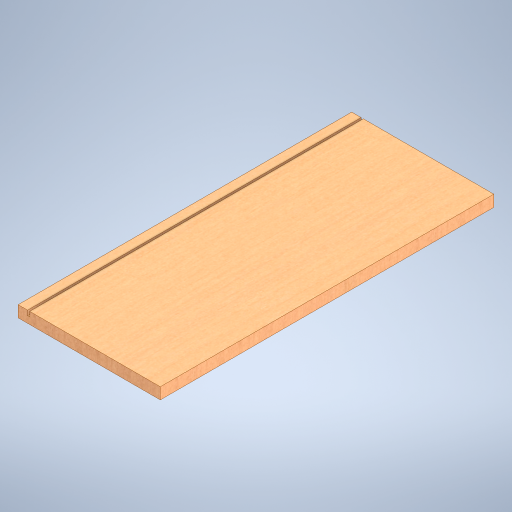
# Autodesk Inventor part: Querseite_Shotclock
Saved by Autodesk Inventor 2024 (Build 280153000, 153)
## iProperties
Created: 2024-03-12
Part Number: Querseite_Shotclock
Material: Holz (Kirsche)
Document SubType Name: Modeling
Designer: haniv
Density: 0.63 g/cm^3
Appearance: Kirsche - natur - schwacher Glanz
Author: haniv
Autodesk Inventor part; units mm, degrees
ref_plane "YZ Plane" through (0, 0, 0) normal (1, 0, 0) x (0, 1, 0)
ref_plane "XZ Plane" through (0, 0, 0) normal (0, 1, 0) x (-1, 0, 0)
ref_plane "XY Plane" through (0, 0, 0) normal (0, 0, 1) x (1, 0, 0)
sketch "Skizze1" plane through (0, 0, 0) normal (0, 0, 1) x (1, 0, 0)
  line L0 (-75, 176) -> (75, 176)
  line L1 (75, 176) -> (75, -176)
  line L2 (75, -176) -> (-75, -176)
  line L3 (-75, -176) -> (-75, 176)
  point P0 (0, 0)
  point P1 (0, 176)
  point P2 (-75, 0)
  dimension "d0" = 150
  dimension "d1" = 352
  constraints: 8 end point, 2 midpoint, 2 parallel, 1 horizontal, 1 horizontal alignment, 1 perpendicular, 1 vertical alignment
  measures "d0" distance of L1.end L2.end
  measures "d1" distance of L0.end L1.end
extrude "Extrusion1" add sketch "Skizze1" along normal blind 12
sketch "Skizze2" plane through (0, 0, 12) normal (0, 0, 1) x (1, 0, 0)
  line L0 (-75, -176) -> (75, -176) projected
  line L1 (75, -176) -> (75, 176) projected
  line L2 (75, 176) -> (-75, 176) projected
  line L3 (-75, 176) -> (-75, -176) projected
  line L4 (75, 176) -> (-75, 176) projected
  line L5 (-65, 176) -> (-62.8, 176)
  line L6 (-62.8, 176) -> (-62.8, -176)
  line L7 (-62.8, -176) -> (-65, -176)
  line L8 (-65, -176) -> (-65, 176)
  point P0 (0, 0)
  dimension "d4" = 10
  dimension "d5" = 2.2
  constraints: 8 end point, 2 parallel, 2 point on line, 1 horizontal, 1 perpendicular
  measures "d4" distance between parallel lines of L8 L3
  measures "d5" distance between parallel lines of L6 L8
extrude "Extrusion2" cut sketch "Skizze2" against normal blind 5 contours L8 L2 L6 L0
